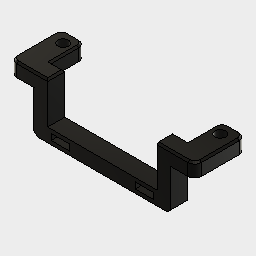
Battery Tray v2 Back (Autodesk Fusion 360 design; units mm, degrees)
Autodesk Fusion 360 part; units mm, degrees
sketch "Sketch1" plane through (0, 0, 0) normal (0, 1, 0) x (1, 0, 0)
  line L0 (-27, 17) -> (-27, 14)
  line L1 (-27, 17) -> (-27, 25)
  line L2 (-25, 27) -> (-22, 27)
  circle A0 centre (-23, 23.5) radius 1.55
  line L3 (-20, 25) -> (-20, 17)
  line L4 (-25, 12) -> (-20, 12)
  line L5 (20, 12) -> (-20, 12)
  line L6 (-20, 17) -> (20, 17)
  line L7 (25, 12) -> (20, 12)
  line L8 (27, 17) -> (27, 14)
  line L9 (27, 17) -> (27, 25)
  line L10 (20, 25) -> (20, 17)
  line L11 (25, 27) -> (22, 27)
  circle A1 centre (23, 23.5) radius 1.55
  line L12 (-20, 17) -> (-20, 12)
  line L13 (20, 17) -> (20, 12)
  line L14 (-20, 17) -> (-16, 17)
  line L15 (-16, 17) -> (-16, 12)
  line L16 (-16, 12) -> (-20, 12)
  line L17 (-20, 12) -> (-20, 17)
  line L18 (20, 17) -> (16, 17)
  line L19 (16, 17) -> (16, 12)
  line L20 (16, 12) -> (20, 12)
  line L21 (20, 12) -> (20, 17)
  arc A2 (-25, 27) -> (-27, 25) centre (-25, 25) ccw
  arc A3 (-20, 25) -> (-22, 27) centre (-22, 25) ccw
  arc A4 (-27, 14) -> (-25, 12) centre (-25, 14) ccw
  arc A5 (25, 12) -> (27, 14) centre (25, 14) ccw
  arc A6 (27, 25) -> (25, 27) centre (25, 25) ccw
  arc A7 (22, 27) -> (20, 25) centre (22, 25) ccw
  dimension "d1" = 5
  dimension "d4" = 4
  dimension "d5" = 5
  dimension "d6" = 4
  dimension "d9" = 2
  measures "d1" distance of L3.end L4.end
  measures "d4" distance of L3.end L14.end
  measures "d5" distance of L3.end L4.end
  measures "d6" distance of L6.end L18.end
  measures "d9" radius of A2
extrude "Extrude3" add sketch "Sketch1" along normal blind 4 contours L0 L1 L2 L3 L4 L12 L17 A2 A3 A4 | L5 L6 L12 L14 L15 L16 L17 | L5 L6 L13 L18 L19 L20 L21 | L7 L8 L9 L10 L11 L13 L21 A5 A6 A7 makes body 1 at (-23.3719, 0, -18.6514) makes body 2 at (23.3719, 0, -18.6514)
extrude "Extrude4" add sketch "Sketch1" against normal blind 8 contours L5 L6 L12 L14 L15 L16 L17 | L5 L6 L13 L18 L19 L20 L21 bodies 1 2
sketch "Sketch2" plane through (0, -8, 0) normal (0, -1, 0) x (1, 0, 0)
  line L0 (-16, -12) -> (-20, -12)
  line L1 (-20, -12) -> (-20, -17)
  line L2 (-20, -17) -> (-16, -17)
  line L3 (-16, -17) -> (-16, -12)
  line L4 (-20, -12) -> (20, -12)
  line L5 (20, -12) -> (20, -17)
  line L6 (20, -17) -> (-20, -17)
  line L7 (-20, -17) -> (-20, -12)
  point P0 (20, -17)
extrude "Extrude5" add sketch "Sketch2" along normal blind 4 bodies 1 2
sketch "Sketch3" plane through (0, 0, -12) normal (0, 0, 1) x (1, 0, 0)
  line L0 (-25, 0) -> (-20, 0)
  line L1 (-20, 0) -> (-20, -12)
  line L2 (-20, -12) -> (20, -12)
  line L3 (20, -12) -> (20, 0)
  line L4 (20, 0) -> (25, 0)
  line L5 (25, 0) -> (25, 4)
  line L6 (25, 4) -> (16, 4)
  line L7 (16, 4) -> (16, -8)
  line L8 (16, -8) -> (-16, -8)
  line L9 (-16, -8) -> (-16, 4)
  line L10 (-16, 4) -> (-25, 4)
  line L11 (-25, 4) -> (-25, 0)
  line L12 (9.6, -9.1) -> (15, -9.1)
  line L13 (-9.6, -9.1) -> (-9.6, -10.9)
  line L14 (15, -10.9) -> (9.6, -10.9)
  line L15 (9.6, -10.9) -> (9.6, -9.1)
  line L16 (-15, -9.1) -> (-9.6, -9.1)
  line L17 (-9.6, -10.9) -> (-15, -10.9)
  line L18 (-15, -10.9) -> (-15, -9.1)
  line L19 (15, -9.1) -> (15, -10.9)
  dimension "d16" = 5.4
  dimension "d17" = 1.8
  dimension "d18" = 5.4
  dimension "d19" = 1.8
  dimension "d20" = 5
  dimension "d21" = 5
  dimension "d22" = 1.1
  dimension "d23" = 1.1
  measures "d16" distance of L14.start L14.end
  measures "d17" distance of L14.start L12.end
  measures "d18" distance of L13.end L17.end
  measures "d19" distance of L13.end L13.start
  measures "d20" distance of L3 L19
  measures "d21" distance of L1 L18
  measures "d22" distance of L8 L16
  measures "d23" distance of L8 L12
extrude "Extrude6" cut sketch "Sketch3" against normal blind 4 contours L12 L14 L15 L19 | L13 L16 L17 L18 bodies 1
chamfer "Chamfer1" distance 1 angle 45 2 edges at (-20, -12, -14.5) (20, -12, -14.5) on bodies 1
chamfer "Chamfer2" distance 0.5 angle 45 18 edges at (-16, 4, -14.5) (-20, 4, -21) (-20.5858, 4, -26.4142) (-23.5, 4, -27) (-26.4142, 4, -26.4142) (-27, 4, -19.5) (-26.4142, 4, -12.5858) (-20.5, 4, -12) (-18, 4, -17) (20.5, 4, -12) (26.4142, 4, -12.5858) (27, 4, -19.5) (26.4142, 4, -26.4142) (23.5, 4, -27) (20.5858, 4, -26.4142) (20, 4, -21) (18, 4, -17) (16, -2, -17) on bodies 1 2
